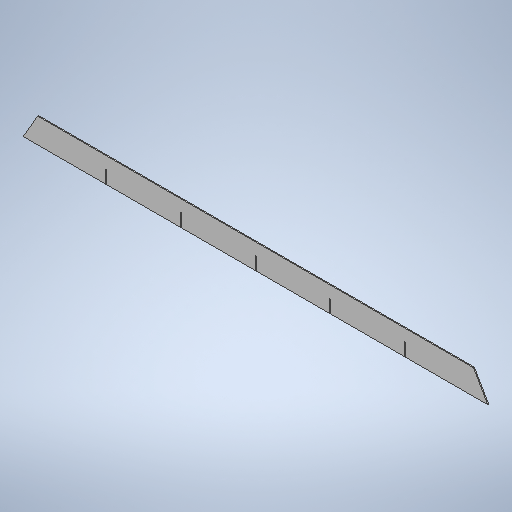
# Autodesk Inventor part: MSC 201 GRID
Saved by Autodesk Inventor 2025 (Build 290162010, 162A)
## iProperties
Created: 2025-01-14
Part Number: MSC 201 GRID
Material: Stainless Steel
Document SubType Name: Sheet Metal
Designer: pokla
Density: 8 g/cm^3
Sheet Metal Rule: AISI304 3mm Die 32
Appearance: Default
Mass: 2760.94 g
Surface Area: 2405.39 cm^2
Volume: 345.117 cm^3
Flat Pattern Width: 8 cm
Flat Pattern Length: 149.238 cm
Flat Pattern Area: 1193.9 cm^2
Sheet Metal Width: 80,000 mm
Sheet Metal Length: 1492,376 mm
Sheet Metal Area: 119390,083 mm^2
Author: pokla
Autodesk Inventor part; units mm, degrees
ref_plane "YZ Plane" through (0, 0, 0) normal (1, 0, 0) x (0, 1, 0)
ref_plane "XZ Plane" through (0, 0, 0) normal (0, 1, 0) x (-1, 0, 0)
ref_plane "XY Plane" through (0, 0, 0) normal (0, 0, 1) x (1, 0, 0)
sketch "Sketch1" plane through (0, 0, 0) normal (0, 1, 0) x (-1, 0, 0)
  line L0 (900, 40) -> (-900, 40)
  line L1 (-900, 40) -> (-900, -40)
  line L2 (-900, -40) -> (900, -40)
  line L3 (900, -40) -> (900, 40)
  line L4 (900, 40) -> (-900, -40) construction
  line L5 (700, 40) -> (746.188, -40)
  line L6 (0, 40) -> (0, -40) construction
  line L7 (-700, 40) -> (-746.188, -40)
  point P0 (0, 0)
  point P1 (0, 0)
  dimension "d0" = 80
  dimension "d1" = 1800
  dimension "d3" = 120
  dimension "d6" = 700
  dimension "d7" = 120
  dimension "d8" = 700
  measures "d0" distance of L2.end L0.start
  measures "d1" distance of L0.start L0.end
  measures "d3" angle of L0 L5
  measures "d6" distance of L6.start L5.start
  measures "d7" angle of L0 L7
  measures "d8" distance of L6.start L7.start
extrude "Plate1" add sketch "Sketch1" along normal mid plane 3 contours L5 L2 L7 L0
sketch "Sketch2" plane through (0, -1.5, 0) normal (0, -1, 0) x (1, 0, 0)
  line L0 (-1.6, -40) -> (1.6, -40)
  line L1 (1.6, -40) -> (1.6, 1)
  line L2 (1.6, 1) -> (-1.6, 1)
  line L3 (-1.6, 1) -> (-1.6, -40)
  line L4 (746.188, -40) -> (-746.188, -40) projected
  point P0 (0, 0)
  point P1 (0, -40)
  dimension "d9" = 3.2
  dimension "d10" = 41
  constraints: 8 end point, 2 midpoint, 2 parallel, 1 horizontal, 1 perpendicular
  measures "d9" distance of L0.start L0.end
  measures "d10" distance of L0.end L1.end
extrude "Extrusion1" cut sketch "Sketch2" against normal through all
pattern_linear "Rectangular Pattern1" count 5 spacing 240 along (1, 0, 0) of "Extrusion1" first direction both ways yes
equation "\"d7\" = d3"
equation "\"d8\" = d6"
equation "\"d2\" = Thickness"
equation "\"BendReliefWidth\" = Thickness"
equation "\"BendReliefDepth\" = 0.5 * Thickness"
equation "\"CornerReliefSize\" = 4 * Thickness"
equation "\"MinimumRemnant\" = 2 * Thickness"
equation "\"TransitionRadius\" = BendRadius"
equation "\"JacobiRadiusSize\" = BendRadius"
equation "\"GapSize\" = Thickness"
equation "\"Thickness\" = 3"
equation "\"BendRadius\" = 5"
body "Solid1"
